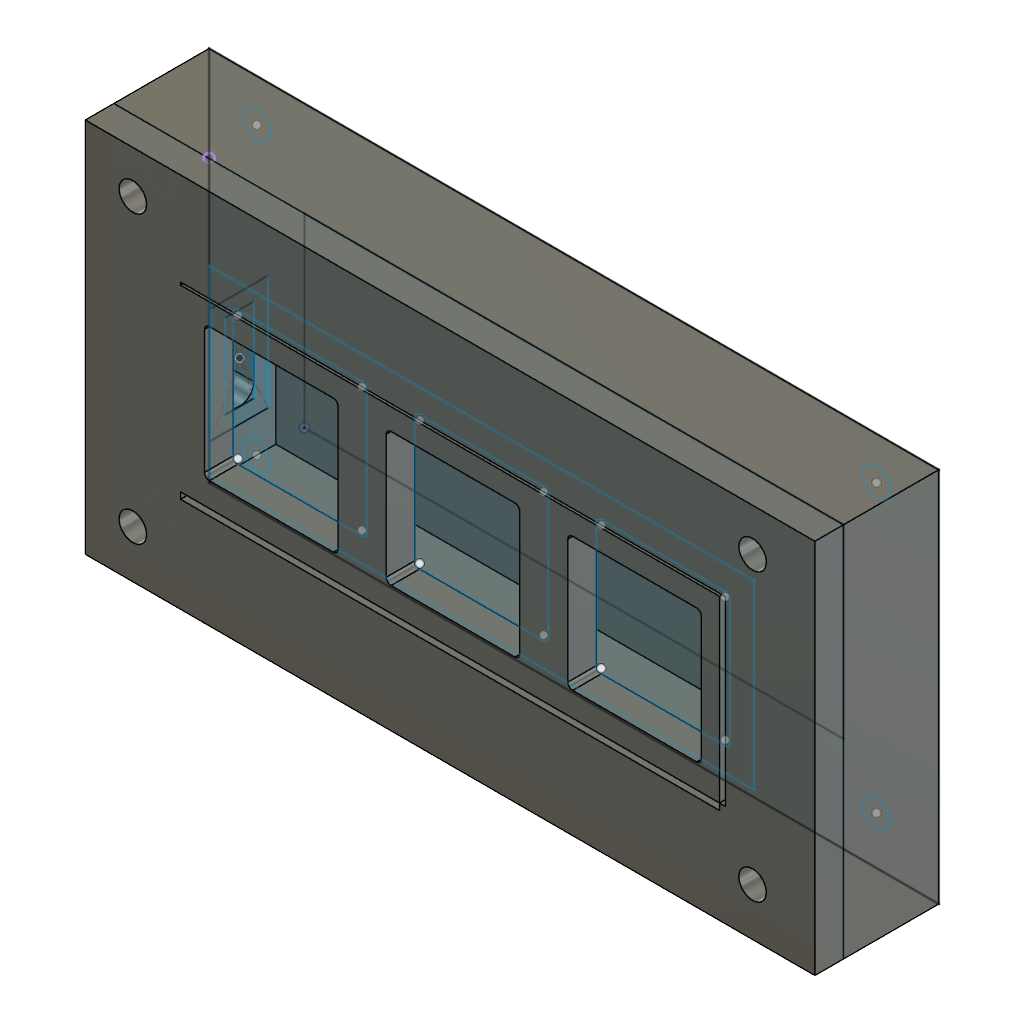
keypad case (Autodesk Fusion 360 design; units mm, degrees)
part number: 2026-09-18-00-52-52-693
Autodesk Fusion 360 part; units mm, degrees
sketch "Sketch1" plane through (0, 0, 0) normal (0, 0, 1) x (1, 0, 0)
  line L0 (0, 0) -> (56.534, 0)
  line L1 (56.534, 0) -> (56.534, 19.45)
  line L2 (56.534, 19.45) -> (0, 19.45)
  line L3 (0, 19.45) -> (0, 0)
  line L4 (-10, -10) -> (66.534, -10)
  line L5 (66.534, -10) -> (66.534, 29.45)
  line L6 (66.534, 29.45) -> (-10, 29.45)
  line L7 (-10, 29.45) -> (-10, -10)
  line L8 (-10, -10) -> (66.534, -10)
  line L9 (66.534, -10) -> (66.534, 29.45)
  line L10 (66.534, 29.45) -> (-10, 29.45)
  line L11 (-10, 29.45) -> (-10, -10)
  circle A0 centre (-5, -5) radius 1.45
  circle A1 centre (-5, 25) radius 1.45
  circle A2 centre (60, 25) radius 1.45
  circle A3 centre (60, -5) radius 1.45
  dimension "d1" = 56.534
  dimension "d2" = 19.45
  dimension "d3" = 10
  dimension "d4" = 10
  dimension "d8" = 2.9
  dimension "d9" = 2.9
  dimension "d10" = 2.9
  dimension "d11" = 2.9
  constraint horizontal L0
  constraint vertical L1
  constraint horizontal L2
  constraint vertical L3
  constraint coincident L0.start L3.end
  measures "d1" distance of L0.start L0.end
  measures "d2" distance of L0.start L2.end
  measures "d8" diameter of A0
  measures "d9" diameter of A1
  measures "d10" diameter of A2
  measures "d11" diameter of A3
extrude "Extrude2" add sketch "Sketch1" along normal blind 3 contours L0 L1 L2 L3 | L4 L5 L6 L7 L8 L9 L10 L11 makes body 1
extrude "Extrude3" add sketch "Sketch1" along normal blind 10 bodies 1
sketch "Sketch3" plane through (0, 0, 10) normal (0, 0, 1) x (1, 0, 0)
  circle A0 centre (60, -5) radius 1.45
  circle A1 centre (-5, 25) radius 1.45
  circle A2 centre (-5, -5) radius 1.45
  circle A3 centre (60, 25) radius 1.45
  line L0 (0, 0) -> (0, 19.45)
  line L1 (0, 19.45) -> (56.534, 19.45)
  line L2 (56.534, 19.45) -> (56.534, 0)
  line L3 (56.534, 0) -> (0, 0)
  line L4 (-10, 29.45) -> (-10, -10)
  line L5 (-10, -10) -> (66.534, -10)
  line L6 (66.534, -10) -> (66.534, 29.45)
  line L7 (66.534, 29.45) -> (-10, 29.45)
  line L8 (3.025, 17.1984) -> (16.025, 17.1984)
  line L9 (3.025, 3.1984) -> (16.025, 3.1984)
  line L10 (2.525, 16.6984) -> (2.525, 3.6984)
  line L11 (16.525, 16.6984) -> (16.525, 3.6984)
  arc A4 (3.025, 17.1984) -> (2.525, 16.6984) centre (3.025, 16.6984) ccw
  arc A5 (16.525, 16.6984) -> (16.025, 17.1984) centre (16.025, 16.6984) ccw
  arc A6 (2.525, 3.6984) -> (3.025, 3.1984) centre (3.025, 3.6984) ccw
  arc A7 (16.025, 3.1984) -> (16.525, 3.6984) centre (16.025, 3.6984) ccw
  line L12 (22.075, 17.1984) -> (35.075, 17.1984)
  line L13 (22.075, 3.1984) -> (35.075, 3.1984)
  line L14 (21.575, 16.6984) -> (21.575, 3.6984)
  line L15 (35.575, 16.6984) -> (35.575, 3.6984)
  arc A8 (22.075, 17.1984) -> (21.575, 16.6984) centre (22.075, 16.6984) ccw
  arc A9 (35.575, 16.6984) -> (35.075, 17.1984) centre (35.075, 16.6984) ccw
  arc A10 (21.575, 3.6984) -> (22.075, 3.1984) centre (22.075, 3.6984) ccw
  arc A11 (35.075, 3.1984) -> (35.575, 3.6984) centre (35.075, 3.6984) ccw
  line L16 (41.125, 17.1984) -> (54.125, 17.1984)
  line L17 (41.125, 3.1984) -> (54.125, 3.1984)
  line L18 (40.625, 16.6984) -> (40.625, 3.6984)
  line L19 (54.625, 16.6984) -> (54.625, 3.6984)
  arc A12 (41.125, 17.1984) -> (40.625, 16.6984) centre (41.125, 16.6984) ccw
  arc A13 (54.625, 16.6984) -> (54.125, 17.1984) centre (54.125, 16.6984) ccw
  arc A14 (40.625, 3.6984) -> (41.125, 3.1984) centre (41.125, 3.6984) ccw
  arc A15 (54.125, 3.1984) -> (54.625, 3.6984) centre (54.125, 3.6984) ccw
  line L20 (0, 0.6734) -> (57.15, 0.6734)
  line L21 (0, 19.7234) -> (57.15, 19.7234)
  line L22 (0, 0.6734) -> (0, 19.7234)
  line L23 (57.15, 0.6734) -> (57.15, 19.7234)
extrude "Extrude4" add sketch "Sketch3" along normal blind 3 separate body contours L0 L1 L2 L20 L22 | L4 L5 L6 L7 makes body 2
sketch "Sketch5" plane through (0, 0, 0) normal (1, 0, 0) x (0, 0, -1)
  line L0 (-3.8, 15.725) -> (-9.8, 15.725)
  line L1 (-9.8, 15.725) -> (-9.8, 3.725)
  line L2 (-9.8, 3.725) -> (-3.8, 3.725)
  line L3 (-3.8, 3.725) -> (-3.8, 15.725)
  line L4 (-3.8, 15.725) -> (-9.8, 3.725) construction
  line L5 (-9.8, 15.725) -> (-3.8, 3.725) construction
  line L6 (-5.3, 14.125) -> (-8.3, 14.125)
  line L7 (-8.3, 14.125) -> (-8.3, 5.325)
  line L8 (-8.3, 5.325) -> (-5.3, 5.325)
  line L9 (-5.3, 5.325) -> (-5.3, 14.125)
  line L10 (-5.3, 14.125) -> (-8.3, 5.325) construction
  line L11 (-8.3, 14.125) -> (-5.3, 5.325) construction
  point P0 (-6.8, 9.725)
  point P1 (-10, 29.45)
  point P2 (-6.8, 9.725)
  dimension "d19" = 6
  dimension "d20" = 12
  dimension "d21" = 19.725
  dimension "d24" = 3
  dimension "d25" = 8.8
  constraint horizontal L0
  constraint perpendicular L0 L1
  constraint parallel L0 L2
  constraint parallel L1 L3
  constraint coincident L4 P2
  constraint coincident L5 P2
  constraint horizontal L6
  constraint perpendicular L6 L7
  constraint parallel L6 L8
  constraint parallel L7 L9
  constraint coincident L10 P2
  constraint coincident L11 P2
  constraint coincident P2 P0
  measures "d19" distance of L1.end L2.end
  measures "d20" distance of L0.end L1.end
  measures "d21" vertical distance of P2 P1
  measures "d24" distance of L7.end L8.end
  measures "d25" distance of L6.end L7.end
extrude "Extrude5" cut sketch "Sketch5" against normal blind 10 contours L6 L7 L8 L9 bodies 1
fillet "Fillet7" radius 1.5 4 edges at (-5, 5.325, 8.3) (-5, 14.125, 8.3) (-5, 5.325, 5.3) (-5, 14.125, 5.3) on bodies 1
sketch "Sketch2" plane through (0, 0, 0) normal (0, 0, 1) x (1, 0, 0)
  point P0 (-5, -5)
  point P1 (-5, 25)
  point P2 (61, 25)
  point P3 (61, -5)
extrude "Extrude1" [suppressed]
equation "d21 = ( 39.45 / 2 ) * 1 mm"
